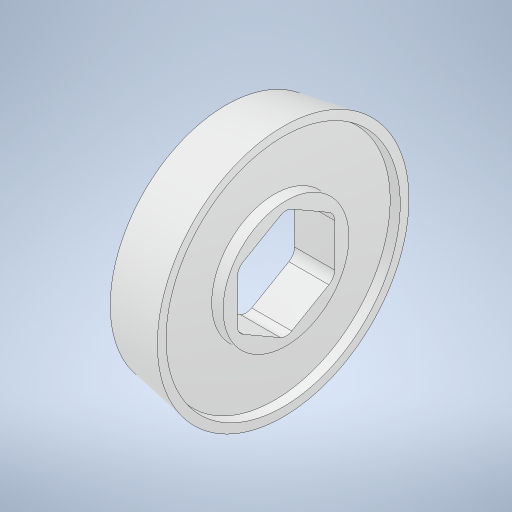
# Autodesk Inventor part: Clutch
Saved by Autodesk Inventor 2023.2 (Build 272271000, 271)
## iProperties
Created: 2024-01-10
Part Number: Clutch
Material: Aluminum 6061
Document SubType Name: Modeling
Designer: Nathan Cai
Mass: 21.1447 g
Surface Area: 60.5598 cm^2
Volume: 7.83136 cm^3
Density: 2.7 g/cm^3
Appearance: Aluminum - Flat
Author: Nathan Cai
Autodesk Inventor part; units mm, degrees
ref_plane "YZ Plane" through (0, 0, 0) normal (1, 0, 0) x (0, 1, 0)
ref_plane "XZ Plane" through (0, 0, 0) normal (0, 1, 0) x (-1, 0, 0)
ref_plane "XY Plane" through (0, 0, 0) normal (0, 0, 1) x (1, 0, 0)
sketch "Sketch1" plane through (0, 0, 0) normal (0, 1, 0) x (-1, 0, 0)
  line L0 (0, 0) -> (3, 0) construction
  line L1 (3, 0) -> (3, -8.5) construction
  line L2 (3, -8.5) -> (0, -8.5) construction
  line L3 (0, -8.5) -> (0, 0) construction
  line L4 (0, -8.5) -> (3, -8.5)
  line L5 (3, -8.5) -> (3, -24)
  line L6 (3, -24) -> (0, -24)
  line L7 (0, -24) -> (0, -8.5)
  line L8 (8.5, -24) -> (-1.5, -24) construction
  line L9 (-1.5, -24) -> (-1.5, -18)
  line L10 (-1.5, -18) -> (8.5, -18)
  line L11 (8.5, -18) -> (8.5, -24)
  line L12 (-1.5, -22) -> (8.5, -20.2367)
  line L13 (-1.5, -20.4769) -> (8.5, -18.7136)
  line L14 (3, -8.5) -> (5, -8.5)
  line L15 (5, -8.5) -> (5, -12.5)
  line L16 (5, -12.5) -> (3, -12.5)
  line L17 (3, -12.5) -> (3, -8.5)
  line L18 (0, -8.5) -> (-2, -8.5)
  line L19 (-2, -8.5) -> (-2, -11)
  line L20 (-2, -11) -> (0, -11)
  line L21 (0, -11) -> (0, -8.5)
  point P0 (3, -18)
  point P1 (0, -18)
  point P2 (0, -20.2124)
  point P3 (3, -19.6834)
  point P4 (3, -12.5)
  point P5 (0, -11)
  dimension "d21" = 3
  dimension "d22" = 8.5
  dimension "d24" = 1.5
  dimension "d25" = 10
  dimension "d26" = 6
  dimension "d27" = 2
  dimension "d28" = 80
  dimension "d29" = 22
  dimension "d30" = 1.5
  dimension "d34" = 2
  dimension "d35" = 4
  dimension "d36" = 2
  dimension "d37" = 2.5
  constraints: 44 end point, 11 parallel, 6 point on line, 5 horizontal, 5 perpendicular
  measures "d21" distance of L1.end L2.end
  measures "d22" distance of L0.end L1.end
  measures "d24" distance between parallel lines of L7 L9
  measures "d25" distance between parallel lines of L9 L11
  measures "d26" distance between parallel lines of L8 L10
  measures "d27" distance from line of L8 L12.start
  measures "d28" angle of L9 L12
  measures "d29" distance from line of L0 L12.start
  measures "d30" distance between parallel lines of L12 L13
  measures "d34" distance of L15.end L16.end
  measures "d35" distance of L14.end L15.end
  measures "d36" distance of L20.end L19.end
  measures "d37" distance of L19.end L18.end
revolve "Revolution1" add sketch "Sketch1" angle 360 about axis through (0, 0, 0) along (-1, 0, 0) contours L4 L5 L10 L7 | L7 L20 L19 L18 | L14 L15 L16 L5 | L10 L5 L13 L7 | L10 L11 L13 L5 | L13 L5 L12 L7 | L7 L12 L9 L13 | L13 L11 L12 L5
sketch "Sketch5" plane through (-3, 0, 0) normal (-1, 0, 0) x (0, 0, 1)
  line L0 (0, 0) -> (-8.5, 0) construction
  circle A0 centre (0, 0) radius 8.5 projected
  line L1 (-8.5, 4.9075) -> (0, 9.815)
  line L2 (0, 9.815) -> (8.5, 4.9075)
  line L3 (8.5, 4.9075) -> (8.5, -4.9075)
  line L4 (8.5, -4.9075) -> (0, -9.815)
  line L5 (0, -9.815) -> (-8.5, -4.9075)
  line L6 (-8.5, -4.9075) -> (-8.5, 4.9075)
  constraints: 14 end point, 1 coincident, 1 horizontal, 1 horizontal alignment, 1 midpoint, 14 other
extrude "Extrusion4" cut sketch "Sketch5" along normal through all both and the other way through all
fillet "Fillet4" radius 2 6 edges at (-1.5, -4.9075, -8.5) (-1.5, 4.9075, -8.5) (-1.5, 9.815, 0) (-1.5, -9.815, 0) (-1.5, -4.9075, 8.5) (-1.5, 4.9075, 8.5)
body "Solid1"
